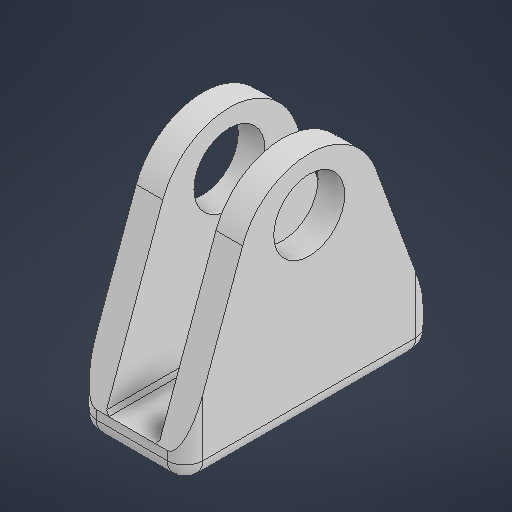
# Autodesk Inventor part: 0.5 in Rod End Bracket (Rough)
Saved by Autodesk Inventor 2026.1 (Build 301233000, 233)
## iProperties
Created: 2026-06-16
Part Number: 0.5 in Rod End Bracket (Rough)
Material: Generic
Document SubType Name: Sheet Metal
Designer: share
Density: 1 g/cm^3
Sheet Metal Rule: Default
Appearance: Default
Author: share
Autodesk Inventor part; units mm, degrees
ref_plane "YZ Plane" through (0, 0, 0) normal (1, 0, 0) x (0, 1, 0)
ref_plane "XZ Plane" through (0, 0, 0) normal (0, 1, 0) x (-1, 0, 0)
ref_plane "XY Plane" through (0, 0, 0) normal (0, 0, 1) x (1, 0, 0)
sketch "Sketch1" plane through (0, 0, 0) normal (0, 1, 0) x (-1, 0, 0)
  line L0 (9.525, 22.225) -> (-9.525, 22.225)
  line L1 (-9.525, 22.225) -> (-9.525, -22.225)
  line L2 (-9.525, -22.225) -> (9.525, -22.225)
  line L3 (9.525, -22.225) -> (9.525, 22.225)
  line L4 (9.525, 22.225) -> (-9.525, -22.225) construction
  line L5 (-9.525, 22.225) -> (9.525, -22.225) construction
  point P0 (0, 0)
  point P1 (-50.8, 0)
  dimension "d0" = 19.05
  dimension "d1" = 44.45
  constraints: 12 end point, 2 midpoint, 2 parallel, 1 horizontal, 1 perpendicular
  measures "d0" distance between parallel lines of L1 L3
  measures "d1" distance between parallel lines of L2 L0
extrude "Base" add sketch "Sketch1" along normal blind 4.7625
sketch "Sketch2" plane through (9.525, 0, 22.225) normal (1, 0, 0) x (0, 0, -1)
  line L0 (0, 0) -> (0, 4.7625) projected
  line L1 (0, 4.7625) -> (10.2968, 32.9347)
  line L2 (0, 4.7625) -> (44.45, 4.7625) projected
  line L3 (34.1532, 32.9347) -> (44.45, 4.7625)
  line L4 (0, 0) -> (44.45, 0) projected
  arc A0 (34.1532, 32.9347) -> (10.2968, 32.9347) centre (22.225, 28.575) ccw
  point P0 (22.225, 0)
  point P1 (22.225, 41.275)
  dimension "d10" = 12.7
  dimension "d12" = 41.275
  constraints: 4 end point, 3 point on circle, 2 tangent, 1 centre point, 1 equal length
  measures "d10" radius of A0
  measures "d12" distance from line of L4 point (22.225, 41.275)
extrude "Vertical 1" add sketch "Sketch2" against normal blind 4.7625
sketch "Sketch3" plane through (-9.525, 0, -22.225) normal (-1, 0, 0) x (0, 0, 1)
  line L0 (44.45, 4.7625) -> (34.1532, 32.9347) projected
  arc A0 (34.1532, 32.9347) -> (10.2968, 32.9347) centre (22.225, 28.575) ccw projected
  line L1 (10.2968, 32.9347) -> (0, 4.7625) projected
  line L2 (44.45, 4.7625) -> (0, 4.7625) projected
  point P0 (22.225, 0)
extrude "Vertical 2" add sketch "Sketch3" against normal blind 4.7625
sketch "Sketch4" plane through (9.525, 0, 22.225) normal (1, 0, 0) x (0, 0, -1)
  arc A0 (34.1532, 32.9347) -> (10.2968, 32.9347) centre (22.225, 28.575) ccw construction
  line L0 (22.225, 41.275) -> (22.225, 0) construction
  circle A1 centre (22.225, 31.75) radius 6.35
  dimension "d17" = 9.525
  dimension "d18" = 12.7
  constraints: 2 end point, 2 point on circle, 1 centre point, 1 point on line, 1 vertical
  measures "d17" distance of A1.centre point (22.225, 41.275)
  measures "d18" diameter of A1
extrude "Bolt Hole" cut sketch "Sketch4" against normal up to surface (19.05 mm away)
fillet "Fillet1" radius 3.175 8 edges at (-9.525, 0, 0) (9.525, 0, 0) (9.525, 2.3813, 22.225) (0, 0, 22.225) (-9.525, 2.3813, 22.225) (9.525, 2.3813, -22.225) (-9.525, 2.3813, -22.225) (0, 0, -22.225)
chamfer "Chamfer1" distance 0.635 angle 45 2 edges at (4.7625, 4.7625, 0) (-4.7625, 4.7625, 0)
equation "\"BendRadius\" = Thickness"
equation "\"BendReliefWidth\" = Thickness"
equation "\"BendReliefDepth\" = 0.5 * Thickness"
equation "\"CornerReliefSize\" = 4 * Thickness"
equation "\"MinimumRemnant\" = 2 * Thickness"
equation "\"TransitionRadius\" = BendRadius"
equation "\"JacobiRadiusSize\" = BendRadius"
equation "\"GapSize\" = Thickness"
equation "\"Thickness\" = 3.048"
body "Solid2"
